Autodesk Inventor part; units mm, degrees
(part 5 of 6)
  line L1822 (91.8375, -60.1869) -> (91.8336, -60.2215) projected
  line L1823 (91.8336, -60.2215) -> (91.829, -60.2562) projected
  line L1824 (91.829, -60.2562) -> (91.8239, -60.2907) projected
  line L1825 (91.8239, -60.2907) -> (91.8181, -60.3251) projected
  line L1826 (91.8181, -60.3251) -> (91.8117, -60.3594) projected
  line L1827 (91.8117, -60.3594) -> (91.8048, -60.3936) projected
  line L1828 (91.8048, -60.3936) -> (91.7972, -60.4277) projected
  line L1829 (91.7972, -60.4277) -> (91.7891, -60.4617) projected
  line L1830 (91.7891, -60.4617) -> (91.7803, -60.4954) projected
  line L1831 (91.7803, -60.4954) -> (91.771, -60.5291) projected
  line L1832 (91.771, -60.5291) -> (91.7611, -60.5626) projected
  line L1833 (91.7611, -60.5626) -> (91.7506, -60.5958) projected
  line L1834 (91.7506, -60.5958) -> (91.7395, -60.6289) projected
  line L1835 (91.7395, -60.6289) -> (91.7279, -60.6618) projected
  line L1836 (91.7279, -60.6618) -> (91.7156, -60.6945) projected
  line L1837 (91.7156, -60.6945) -> (91.7028, -60.727) projected
  line L1838 (91.7028, -60.727) -> (91.6895, -60.7593) projected
  line L1839 (91.6895, -60.7593) -> (91.6756, -60.7913) projected
  line L1840 (91.6756, -60.7913) -> (91.6611, -60.823) projected
  line L1841 (91.6611, -60.823) -> (91.6461, -60.8546) projected
  line L1842 (91.6461, -60.8546) -> (91.6305, -60.8858) projected
  line L1843 (91.6305, -60.8858) -> (91.6144, -60.9168) projected
  line L1844 (91.6144, -60.9168) -> (91.5977, -60.9474) projected
  line L1845 (91.5977, -60.9474) -> (91.5805, -60.9778) projected
  line L1846 (91.5805, -60.9778) -> (91.5628, -61.0079) projected
  line L1847 (91.5628, -61.0079) -> (91.5446, -61.0376) projected
  line L1848 (91.5446, -61.0376) -> (91.5258, -61.0671) projected
  line L1849 (91.5258, -61.0671) -> (91.5066, -61.0962) projected
  line L1850 (91.5066, -61.0962) -> (91.4868, -61.125) projected
  line L1851 (91.4868, -61.125) -> (91.4665, -61.1534) projected
  line L1852 (91.4665, -61.1534) -> (91.4458, -61.1814) projected
  line L1853 (91.4458, -61.1814) -> (91.4245, -61.2091) projected
  line L1854 (91.4245, -61.2091) -> (91.4028, -61.2364) projected
  line L1855 (91.4028, -61.2364) -> (91.3806, -61.2634) projected
  line L1856 (91.3806, -61.2634) -> (91.3579, -61.2899) projected
  line L1857 (91.3579, -61.2899) -> (91.3348, -61.3161) projected
  line L1858 (91.3348, -61.3161) -> (91.3112, -61.3418) projected
  line L1859 (91.3112, -61.3418) -> (91.2872, -61.3671) projected
  line L1860 (91.2872, -61.3671) -> (91.2627, -61.392) projected
  line L1861 (91.2627, -61.392) -> (91.2378, -61.4165) projected
  line L1862 (91.2378, -61.4165) -> (91.2125, -61.4405) projected
  line L1863 (91.2125, -61.4405) -> (91.1867, -61.4641) projected
  line L1864 (91.1867, -61.4641) -> (91.1606, -61.4872) projected
  line L1865 (91.1606, -61.4872) -> (91.1341, -61.5099) projected
  line L1866 (91.1341, -61.5099) -> (91.1071, -61.5321) projected
  line L1867 (91.1071, -61.5321) -> (91.0798, -61.5538) projected
  line L1868 (91.0798, -61.5538) -> (91.0521, -61.5751) projected
  line L1869 (91.0521, -61.5751) -> (91.0241, -61.5958) projected
  line L1870 (91.0241, -61.5958) -> (90.9956, -61.6161) projected
  line L1871 (90.9956, -61.6161) -> (90.9669, -61.6359) projected
  line L1872 (90.9669, -61.6359) -> (90.9378, -61.6551) projected
  line L1873 (90.9378, -61.6551) -> (90.9083, -61.6739) projected
  line L1874 (90.9083, -61.6739) -> (90.8786, -61.6921) projected
  line L1875 (90.8786, -61.6921) -> (90.8485, -61.7099) projected
  line L1876 (90.8485, -61.7099) -> (90.8181, -61.727) projected
  line L1877 (90.8181, -61.727) -> (90.7874, -61.7437) projected
  line L1878 (90.7874, -61.7437) -> (90.7565, -61.7598) projected
  line L1879 (90.7565, -61.7598) -> (90.7252, -61.7754) projected
  line L1880 (90.7252, -61.7754) -> (90.6937, -61.7904) projected
  line L1881 (90.6937, -61.7904) -> (90.662, -61.8049) projected
  line L1882 (90.662, -61.8049) -> (90.6299, -61.8188) projected
  line L1883 (90.6299, -61.8188) -> (90.5977, -61.8322) projected
  line L1884 (90.5977, -61.8322) -> (90.5652, -61.845) projected
  line L1885 (90.5652, -61.845) -> (90.5325, -61.8572) projected
  line L1886 (90.5325, -61.8572) -> (90.4996, -61.8688) projected
  line L1887 (90.4996, -61.8688) -> (90.4665, -61.8799) projected
  line L1888 (90.4665, -61.8799) -> (90.4332, -61.8904) projected
  line L1889 (90.4332, -61.8904) -> (90.3998, -61.9003) projected
  line L1890 (90.3998, -61.9003) -> (90.3661, -61.9097) projected
  line L1891 (90.3661, -61.9097) -> (90.3323, -61.9184) projected
  line L1892 (90.3323, -61.9184) -> (90.2984, -61.9265) projected
  line L1893 (90.2984, -61.9265) -> (90.2643, -61.9341) projected
  line L1894 (90.2643, -61.9341) -> (90.2301, -61.9411) projected
  line L1895 (90.2301, -61.9411) -> (90.1958, -61.9474) projected
  line L1896 (90.1958, -61.9474) -> (90.1614, -61.9532) projected
  line L1897 (90.1614, -61.9532) -> (90.1268, -61.9583) projected
  line L1898 (90.1268, -61.9583) -> (90.0922, -61.9629) projected
  line L1899 (90.0922, -61.9629) -> (90.0575, -61.9668) projected
  line L1900 (90.0575, -61.9668) -> (90.0228, -61.9702) projected
  line L1901 (90.0228, -61.9702) -> (89.988, -61.9729) projected
  line L1902 (89.988, -61.9729) -> (89.9532, -61.9751) projected
  line L1903 (89.9532, -61.9751) -> (89.9183, -61.9766) projected
  line L1904 (89.9183, -61.9766) -> (89.8834, -61.9775) projected
  line L1905 (89.8834, -61.9775) -> (89.8485, -61.9778) projected
  line L1906 (89.8485, -61.9778) -> (89.8136, -61.9775) projected
  line L1907 (89.8136, -61.9775) -> (89.7787, -61.9766) projected
  line L1908 (89.7787, -61.9766) -> (89.7438, -61.9751) projected
  line L1909 (89.7438, -61.9751) -> (89.709, -61.9729) projected
  line L1910 (89.709, -61.9729) -> (89.6742, -61.9702) projected
  line L1911 (89.6742, -61.9702) -> (89.6394, -61.9668) projected
  line L1912 (89.6394, -61.9668) -> (89.6047, -61.9629) projected
  line L1913 (89.6047, -61.9629) -> (89.5701, -61.9583) projected
  line L1914 (89.5701, -61.9583) -> (89.5356, -61.9532) projected
  line L1915 (89.5356, -61.9532) -> (89.5012, -61.9474) projected
  line L1916 (89.5012, -61.9474) -> (89.4669, -61.9411) projected
  line L1917 (89.4669, -61.9411) -> (89.4327, -61.9341) projected
  line L1918 (89.4327, -61.9341) -> (89.3986, -61.9265) projected
  line L1919 (89.3986, -61.9265) -> (89.3646, -61.9184) projected
  line L1920 (89.3646, -61.9184) -> (89.3308, -61.9097) projected
  line L1921 (89.3308, -61.9097) -> (89.2972, -61.9003) projected
  line L1922 (89.2972, -61.9003) -> (89.2637, -61.8904) projected
  line L1923 (89.2637, -61.8904) -> (89.2305, -61.8799) projected
  line L1924 (89.2305, -61.8799) -> (89.1973, -61.8688) projected
  line L1925 (89.1973, -61.8688) -> (89.1644, -61.8572) projected
  line L1926 (89.1644, -61.8572) -> (89.1317, -61.845) projected
  line L1927 (89.1317, -61.845) -> (89.0993, -61.8322) projected
  line L1928 (89.0993, -61.8322) -> (89.067, -61.8188) projected
  line L1929 (89.067, -61.8188) -> (89.035, -61.8049) projected
  line L1930 (89.035, -61.8049) -> (89.0032, -61.7904) projected
  line L1931 (89.0032, -61.7904) -> (88.9717, -61.7754) projected
  line L1932 (88.9717, -61.7754) -> (88.9405, -61.7598) projected
  line L1933 (88.9405, -61.7598) -> (88.9095, -61.7437) projected
  line L1934 (88.9095, -61.7437) -> (88.8789, -61.727) projected
  line L1935 (88.8789, -61.727) -> (88.8485, -61.7099) projected
  line L1936 (88.8485, -61.7099) -> (88.8184, -61.6921) projected
  line L1937 (88.8184, -61.6921) -> (88.7886, -61.6739) projected
  line L1938 (88.7886, -61.6739) -> (88.7592, -61.6551) projected
  line L1939 (88.7592, -61.6551) -> (88.7301, -61.6359) projected
  line L1940 (88.7301, -61.6359) -> (88.7013, -61.6161) projected
  line L1941 (88.7013, -61.6161) -> (88.6729, -61.5958) projected
  line L1942 (88.6729, -61.5958) -> (88.6449, -61.5751) projected
  line L1943 (88.6449, -61.5751) -> (88.6172, -61.5538) projected
  line L1944 (88.6172, -61.5538) -> (88.5898, -61.5321) projected
  line L1945 (88.5898, -61.5321) -> (88.5629, -61.5099) projected
  line L1946 (88.5629, -61.5099) -> (88.5364, -61.4872) projected
  line L1947 (88.5364, -61.4872) -> (88.5102, -61.4641) projected
  line L1948 (88.5102, -61.4641) -> (88.4845, -61.4405) projected
  line L1949 (88.4845, -61.4405) -> (88.4592, -61.4165) projected
  line L1950 (88.4592, -61.4165) -> (88.4343, -61.392) projected
  line L1951 (88.4343, -61.392) -> (88.4098, -61.3671) projected
  line L1952 (88.4098, -61.3671) -> (88.3858, -61.3418) projected
  line L1953 (88.3858, -61.3418) -> (88.3622, -61.3161) projected
  line L1954 (88.3622, -61.3161) -> (88.3391, -61.2899) projected
  line L1955 (88.3391, -61.2899) -> (88.3164, -61.2634) projected
  line L1956 (88.3164, -61.2634) -> (88.2942, -61.2364) projected
  line L1957 (88.2942, -61.2364) -> (88.2725, -61.2091) projected
  line L1958 (88.2725, -61.2091) -> (88.2512, -61.1814) projected
  line L1959 (88.2512, -61.1814) -> (88.2305, -61.1534) projected
  line L1960 (88.2305, -61.1534) -> (88.2102, -61.125) projected
  line L1961 (88.2102, -61.125) -> (88.1904, -61.0962) projected
  line L1962 (88.1904, -61.0962) -> (88.1711, -61.0671) projected
  line L1963 (88.1711, -61.0671) -> (88.1524, -61.0376) projected
  line L1964 (88.1524, -61.0376) -> (88.1342, -61.0079) projected
  line L1965 (88.1342, -61.0079) -> (88.1164, -60.9778) projected
  line L1966 (88.1164, -60.9778) -> (88.0992, -60.9474) projected
  line L1967 (88.0992, -60.9474) -> (88.0826, -60.9168) projected
  line L1968 (88.0826, -60.9168) -> (88.0665, -60.8858) projected
  line L1969 (88.0665, -60.8858) -> (88.0509, -60.8546) projected
  line L1970 (88.0509, -60.8546) -> (88.0359, -60.823) projected
  line L1971 (88.0359, -60.823) -> (88.0214, -60.7913) projected
  line L1972 (88.0214, -60.7913) -> (88.0075, -60.7593) projected
  line L1973 (88.0075, -60.7593) -> (87.9941, -60.727) projected
  line L1974 (87.9941, -60.727) -> (87.9813, -60.6945) projected
  line L1975 (87.9813, -60.6945) -> (87.9691, -60.6618) projected
  line L1976 (87.9691, -60.6618) -> (87.9575, -60.6289) projected
  line L1977 (87.9575, -60.6289) -> (87.9464, -60.5958) projected
  line L1978 (87.9464, -60.5958) -> (87.9359, -60.5626) projected
  line L1979 (87.9359, -60.5626) -> (87.926, -60.5291) projected
  line L1980 (87.926, -60.5291) -> (87.9166, -60.4954) projected
  line L1981 (87.9166, -60.4954) -> (87.9079, -60.4617) projected
  line L1982 (87.9079, -60.4617) -> (87.8997, -60.4277) projected
  line L1983 (87.8997, -60.4277) -> (87.8922, -60.3936) projected
  line L1984 (87.8922, -60.3936) -> (87.8852, -60.3594) projected
  line L1985 (87.8852, -60.3594) -> (87.8789, -60.3251) projected
  line L1986 (87.8789, -60.3251) -> (87.8731, -60.2907) projected
  line L1987 (87.8731, -60.2907) -> (87.868, -60.2562) projected
  line L1988 (87.868, -60.2562) -> (87.8634, -60.2215) projected
  line L1989 (87.8634, -60.2215) -> (87.8594, -60.1869) projected
  line L1990 (87.8594, -60.1869) -> (87.8561, -60.1521) projected
  line L1991 (87.8561, -60.1521) -> (87.8534, -60.1173) projected
  line L1992 (87.8534, -60.1173) -> (87.8512, -60.0825) projected
  line L1993 (87.8512, -60.0825) -> (87.8497, -60.0476) projected
  line L1994 (87.8497, -60.0476) -> (87.8488, -60.0127) projected
  line L1995 (87.8488, -60.0127) -> (87.8485, -59.9778) projected
  line L1996 (87.8485, -59.9778) -> (87.8488, -59.9429) projected
  line L1997 (87.8488, -59.9429) -> (87.8497, -59.908) projected
  line L1998 (87.8497, -59.908) -> (87.8512, -59.8731) projected
  line L1999 (87.8512, -59.8731) -> (87.8534, -59.8383) projected
  line L2000 (87.8534, -59.8383) -> (87.8561, -59.8035) projected
  line L2001 (87.8561, -59.8035) -> (87.8594, -59.7688) projected
  line L2002 (87.8594, -59.7688) -> (87.8634, -59.7341) projected
  line L2003 (87.8634, -59.7341) -> (87.868, -59.6995) projected
  line L2004 (87.868, -59.6995) -> (87.8731, -59.6649) projected
  line L2005 (87.8731, -59.6649) -> (87.8789, -59.6305) projected
  line L2006 (87.8789, -59.6305) -> (87.8852, -59.5962) projected
  line L2007 (87.8852, -59.5962) -> (87.8922, -59.562) projected
  line L2008 (87.8922, -59.562) -> (87.8997, -59.5279) projected
  line L2009 (87.8997, -59.5279) -> (87.9079, -59.494) projected
  line L2010 (87.9079, -59.494) -> (87.9166, -59.4602) projected
  line L2011 (87.9166, -59.4602) -> (87.926, -59.4265) projected
  line L2012 (87.926, -59.4265) -> (87.9359, -59.3931) projected
  line L2013 (87.9359, -59.3931) -> (87.9464, -59.3598) projected
  line L2014 (87.9464, -59.3598) -> (87.9575, -59.3267) projected
  line L2015 (87.9575, -59.3267) -> (87.9691, -59.2938) projected
  line L2016 (87.9691, -59.2938) -> (87.9813, -59.2611) projected
  line L2017 (87.9813, -59.2611) -> (87.9941, -59.2286) projected
  line L2018 (87.9941, -59.2286) -> (88.0075, -59.1963) projected
  line L2019 (88.0075, -59.1963) -> (88.0214, -59.1643) projected
  line L2020 (88.0214, -59.1643) -> (88.0359, -59.1326) projected
  line L2021 (88.0359, -59.1326) -> (88.0509, -59.1011) projected
  line L2022 (88.0509, -59.1011) -> (88.0665, -59.0698) projected
  line L2023 (88.0665, -59.0698) -> (88.0826, -59.0389) projected
  line L2024 (88.0826, -59.0389) -> (88.0992, -59.0082) projected
  line L2025 (88.0992, -59.0082) -> (88.1164, -58.9778) projected
  line L2026 (88.1164, -58.9778) -> (88.1342, -58.9477) projected
  line L2027 (88.1342, -58.9477) -> (88.1524, -58.918) projected
  line L2028 (88.1524, -58.918) -> (88.1711, -58.8885) projected
  line L2029 (88.1711, -58.8885) -> (88.1904, -58.8594) projected
  line L2030 (88.1904, -58.8594) -> (88.2102, -58.8307) projected
  line L2031 (88.2102, -58.8307) -> (88.2305, -58.8022) projected
  line L2032 (88.2305, -58.8022) -> (88.2512, -58.7742) projected
  line L2033 (88.2512, -58.7742) -> (88.2725, -58.7465) projected
  line L2034 (88.2725, -58.7465) -> (88.2942, -58.7192) projected
  line L2035 (88.2942, -58.7192) -> (88.3164, -58.6922) projected
  line L2036 (88.3164, -58.6922) -> (88.3391, -58.6657) projected
  line L2037 (88.3391, -58.6657) -> (88.3622, -58.6396) projected
  line L2038 (88.3622, -58.6396) -> (88.3858, -58.6138) projected
  line L2039 (88.3858, -58.6138) -> (88.4098, -58.5885) projected
  line L2040 (88.4098, -58.5885) -> (88.4343, -58.5636) projected
  line L2041 (88.4343, -58.5636) -> (88.4592, -58.5391) projected
  line L2042 (88.4592, -58.5391) -> (88.4845, -58.5151) projected
  line L2043 (88.4845, -58.5151) -> (88.5102, -58.4915) projected
  line L2044 (88.5102, -58.4915) -> (88.5364, -58.4684) projected
  line L2045 (88.5364, -58.4684) -> (88.5629, -58.4457) projected
  line L2046 (88.5629, -58.4457) -> (88.5898, -58.4235) projected
  line L2047 (88.5898, -58.4235) -> (88.6172, -58.4018) projected
  line L2048 (88.6172, -58.4018) -> (88.6449, -58.3805) projected
  line L2049 (88.6449, -58.3805) -> (88.6729, -58.3598) projected
  line L2050 (88.6729, -58.3598) -> (88.7013, -58.3395) projected
  line L2051 (88.7013, -58.3395) -> (88.7301, -58.3197) projected
  line L2052 (88.7301, -58.3197) -> (88.7592, -58.3005) projected
  line L2053 (88.7592, -58.3005) -> (88.7886, -58.2817) projected
  line L2054 (88.7886, -58.2817) -> (88.8184, -58.2635) projected
  line L2055 (88.8184, -58.2635) -> (88.8485, -58.2458) projected
  line L2056 (88.8485, -58.2458) -> (88.8789, -58.2286) projected
  line L2057 (88.8789, -58.2286) -> (88.9095, -58.2119) projected
  line L2058 (88.9095, -58.2119) -> (88.9405, -58.1958) projected
  line L2059 (88.9405, -58.1958) -> (88.9717, -58.1802) projected
  line L2060 (88.9717, -58.1802) -> (89.0032, -58.1652) projected
  line L2061 (89.0032, -58.1652) -> (89.035, -58.1507) projected
  line L2062 (89.035, -58.1507) -> (89.067, -58.1368) projected
  line L2063 (89.067, -58.1368) -> (89.0993, -58.1234) projected
  line L2064 (89.0993, -58.1234) -> (89.1317, -58.1107) projected
  line L2065 (89.1317, -58.1107) -> (89.1644, -58.0984) projected
  line L2066 (89.1644, -58.0984) -> (89.1973, -58.0868) projected
  line L2067 (89.1973, -58.0868) -> (89.2305, -58.0757) projected
  line L2068 (89.2305, -58.0757) -> (89.2637, -58.0652) projected
  line L2069 (89.2637, -58.0652) -> (89.2972, -58.0553) projected
  line L2070 (89.2972, -58.0553) -> (89.3308, -58.046) projected
  line L2071 (89.3308, -58.046) -> (89.3646, -58.0372) projected
  line L2072 (89.3646, -58.0372) -> (89.3986, -58.0291) projected
  line L2073 (89.3986, -58.0291) -> (89.4327, -58.0215) projected
  line L2074 (89.4327, -58.0215) -> (89.4669, -58.0146) projected
  line L2075 (89.4669, -58.0146) -> (89.5012, -58.0082) projected
  line L2076 (89.5012, -58.0082) -> (89.5356, -58.0024) projected
  line L2077 (89.5356, -58.0024) -> (89.5701, -57.9973) projected
  line L2078 (89.5701, -57.9973) -> (89.6047, -57.9927) projected
  line L2079 (89.6047, -57.9927) -> (89.6394, -57.9888) projected
  line L2080 (89.6394, -57.9888) -> (89.6742, -57.9854) projected
  line L2081 (89.6742, -57.9854) -> (89.709, -57.9827) projected
  line L2082 (89.709, -57.9827) -> (89.7438, -57.9806) projected
  line L2083 (89.7438, -57.9806) -> (89.7787, -57.979) projected
  line L2084 (89.7787, -57.979) -> (89.8136, -57.9781) projected
  line L2085 (89.8136, -57.9781) -> (89.8485, -57.9778) projected
  line L2086 (89.8485, -57.9778) -> (89.8834, -57.9781) projected
  line L2087 (89.8834, -57.9781) -> (89.9183, -57.979) projected
  line L2088 (89.9183, -57.979) -> (89.9532, -57.9806) projected
  line L2089 (89.9532, -57.9806) -> (89.988, -57.9827) projected
  line L2090 (89.988, -57.9827) -> (90.0228, -57.9854) projected
  line L2091 (90.0228, -57.9854) -> (90.0575, -57.9888) projected
  line L2092 (90.0575, -57.9888) -> (90.0922, -57.9927) projected
  line L2093 (90.0922, -57.9927) -> (90.1268, -57.9973) projected
  line L2094 (90.1268, -57.9973) -> (90.1614, -58.0024) projected
  line L2095 (90.1614, -58.0024) -> (90.1958, -58.0082) projected
  line L2096 (90.1958, -58.0082) -> (90.2301, -58.0146) projected
  line L2097 (90.2301, -58.0146) -> (90.2643, -58.0215) projected
  line L2098 (90.2643, -58.0215) -> (90.2984, -58.0291) projected
  line L2099 (90.2984, -58.0291) -> (90.3323, -58.0372) projected
  line L2100 (90.3323, -58.0372) -> (90.3661, -58.046) projected
  line L2101 (90.3661, -58.046) -> (90.3998, -58.0553) projected
  line L2102 (90.3998, -58.0553) -> (90.4332, -58.0652) projected
  line L2103 (90.4332, -58.0652) -> (90.4665, -58.0757) projected
  line L2104 (90.4665, -58.0757) -> (90.4996, -58.0868) projected
  line L2105 (90.4996, -58.0868) -> (90.5325, -58.0984) projected
  line L2106 (90.5325, -58.0984) -> (90.5652, -58.1107) projected
  line L2107 (90.5652, -58.1107) -> (90.5977, -58.1234) projected
  line L2108 (90.5977, -58.1234) -> (90.6299, -58.1368) projected
  line L2109 (90.6299, -58.1368) -> (90.662, -58.1507) projected
  line L2110 (90.662, -58.1507) -> (90.6937, -58.1652) projected
  line L2111 (90.6937, -58.1652) -> (90.7252, -58.1802) projected
  line L2112 (90.7252, -58.1802) -> (90.7565, -58.1958) projected
  line L2113 (90.7565, -58.1958) -> (90.7874, -58.2119) projected
  line L2114 (90.7874, -58.2119) -> (90.8181, -58.2286) projected
  line L2115 (90.8181, -58.2286) -> (90.8485, -58.2458) projected
  line L2116 (90.8485, -58.2458) -> (90.8786, -58.2635) projected
  line L2117 (90.8786, -58.2635) -> (90.9083, -58.2817) projected
  line L2118 (90.9083, -58.2817) -> (90.9378, -58.3005) projected
  line L2119 (90.9378, -58.3005) -> (90.9669, -58.3197) projected
  line L2120 (90.9669, -58.3197) -> (90.9956, -58.3395) projected
  line L2121 (90.9956, -58.3395) -> (91.0241, -58.3598) projected
  line L2122 (91.0241, -58.3598) -> (91.0521, -58.3805) projected
  line L2123 (91.0521, -58.3805) -> (91.0798, -58.4018) projected
  line L2124 (91.0798, -58.4018) -> (91.1071, -58.4235) projected
  line L2125 (91.1071, -58.4235) -> (91.1341, -58.4457) projected
  line L2126 (91.1341, -58.4457) -> (91.1606, -58.4684) projected
  line L2127 (91.1606, -58.4684) -> (91.1867, -58.4915) projected
  line L2128 (91.1867, -58.4915) -> (91.2125, -58.5151) projected
  line L2129 (91.2125, -58.5151) -> (91.2378, -58.5391) projected
  line L2130 (91.2378, -58.5391) -> (91.2627, -58.5636) projected
  line L2131 (91.2627, -58.5636) -> (91.2872, -58.5885) projected
  line L2132 (91.2872, -58.5885) -> (91.3112, -58.6138) projected
  line L2133 (91.3112, -58.6138) -> (91.3348, -58.6396) projected
  line L2134 (91.3348, -58.6396) -> (91.3579, -58.6657) projected
  line L2135 (91.3579, -58.6657) -> (91.3806, -58.6922) projected
  line L2136 (91.3806, -58.6922) -> (91.4028, -58.7192) projected
  line L2137 (91.4028, -58.7192) -> (91.4245, -58.7465) projected
  line L2138 (91.4245, -58.7465) -> (91.4458, -58.7742) projected
  line L2139 (91.4458, -58.7742) -> (91.4665, -58.8022) projected
  line L2140 (91.4665, -58.8022) -> (91.4868, -58.8307) projected
  line L2141 (91.4868, -58.8307) -> (91.5066, -58.8594) projected
  line L2142 (91.5066, -58.8594) -> (91.5258, -58.8885) projected
  line L2143 (91.5258, -58.8885) -> (91.5446, -58.918) projected
  line L2144 (91.5446, -58.918) -> (91.5628, -58.9477) projected
  line L2145 (91.5628, -58.9477) -> (91.5805, -58.9778) projected
  line L2146 (91.5805, -58.9778) -> (91.5977, -59.0082) projected
  line L2147 (91.5977, -59.0082) -> (91.6144, -59.0389) projected
  line L2148 (91.6144, -59.0389) -> (91.6305, -59.0698) projected
  line L2149 (91.6305, -59.0698) -> (91.6461, -59.1011) projected
  line L2150 (91.6461, -59.1011) -> (91.6611, -59.1326) projected
  line L2151 (91.6611, -59.1326) -> (91.6756, -59.1643) projected
  line L2152 (91.6756, -59.1643) -> (91.6895, -59.1963) projected
  line L2153 (91.6895, -59.1963) -> (91.7028, -59.2286) projected
  line L2154 (91.7028, -59.2286) -> (91.7156, -59.2611) projected
  line L2155 (91.7156, -59.2611) -> (91.7279, -59.2938) projected
  line L2156 (91.7279, -59.2938) -> (91.7395, -59.3267) projected
  line L2157 (91.7395, -59.3267) -> (91.7506, -59.3598) projected
  line L2158 (91.7506, -59.3598) -> (91.7611, -59.3931) projected
  line L2159 (91.7611, -59.3931) -> (91.771, -59.4265) projected
  line L2160 (91.771, -59.4265) -> (91.7803, -59.4602) projected
  line L2161 (91.7803, -59.4602) -> (91.7891, -59.494) projected
  line L2162 (91.7891, -59.494) -> (91.7972, -59.5279) projected
  line L2163 (91.7972, -59.5279) -> (91.8048, -59.562) projected
  line L2164 (91.8048, -59.562) -> (91.8117, -59.5962) projected
  line L2165 (91.8117, -59.5962) -> (91.8181, -59.6305) projected
  line L2166 (91.8181, -59.6305) -> (91.8239, -59.6649) projected
  line L2167 (91.8239, -59.6649) -> (91.829, -59.6995) projected
  line L2168 (91.829, -59.6995) -> (91.8336, -59.7341) projected
  line L2169 (91.8336, -59.7341) -> (91.8375, -59.7688) projected
  line L2170 (91.8375, -59.7688) -> (91.8409, -59.8035) projected
  line L2171 (91.8409, -59.8035) -> (91.8436, -59.8383) projected
  line L2172 (91.8436, -59.8383) -> (91.8457, -59.8731) projected
  line L2173 (91.8457, -59.8731) -> (91.8473, -59.908) projected
  line L2174 (91.8473, -59.908) -> (91.8482, -59.9429) projected
  line L2175 (91.8482, -59.9429) -> (91.8485, -59.9778) projected
  line L2176 (-88.1514, -59.9778) -> (-88.1517, -60.0127) projected
  line L2177 (-88.1517, -60.0127) -> (-88.1526, -60.0476) projected
  line L2178 (-88.1526, -60.0476) -> (-88.1542, -60.0825) projected
  line L2179 (-88.1542, -60.0825) -> (-88.1563, -60.1173) projected
  line L2180 (-88.1563, -60.1173) -> (-88.159, -60.1521) projected
  line L2181 (-88.159, -60.1521) -> (-88.1624, -60.1869) projected
  line L2182 (-88.1624, -60.1869) -> (-88.1663, -60.2215) projected
  line L2183 (-88.1663, -60.2215) -> (-88.1709, -60.2562) projected
  line L2184 (-88.1709, -60.2562) -> (-88.176, -60.2907) projected
  line L2185 (-88.176, -60.2907) -> (-88.1818, -60.3251) projected
  line L2186 (-88.1818, -60.3251) -> (-88.1882, -60.3594) projected
  line L2187 (-88.1882, -60.3594) -> (-88.1951, -60.3936) projected
  line L2188 (-88.1951, -60.3936) -> (-88.2027, -60.4277) projected
  line L2189 (-88.2027, -60.4277) -> (-88.2108, -60.4617) projected
  line L2190 (-88.2108, -60.4617) -> (-88.2196, -60.4954) projected
  line L2191 (-88.2196, -60.4954) -> (-88.2289, -60.5291) projected
  line L2192 (-88.2289, -60.5291) -> (-88.2388, -60.5626) projected
  line L2193 (-88.2388, -60.5626) -> (-88.2493, -60.5958) projected
  line L2194 (-88.2493, -60.5958) -> (-88.2604, -60.6289) projected
  line L2195 (-88.2604, -60.6289) -> (-88.272, -60.6618) projected
  line L2196 (-88.272, -60.6618) -> (-88.2843, -60.6945) projected
  line L2197 (-88.2843, -60.6945) -> (-88.297, -60.727) projected
  line L2198 (-88.297, -60.727) -> (-88.3104, -60.7593) projected
  line L2199 (-88.3104, -60.7593) -> (-88.3243, -60.7913) projected
  line L2200 (-88.3243, -60.7913) -> (-88.3388, -60.823) projected
  line L2201 (-88.3388, -60.823) -> (-88.3538, -60.8546) projected
  line L2202 (-88.3538, -60.8546) -> (-88.3694, -60.8858) projected
  line L2203 (-88.3694, -60.8858) -> (-88.3855, -60.9168) projected
  line L2204 (-88.3855, -60.9168) -> (-88.4022, -60.9474) projected
  line L2205 (-88.4022, -60.9474) -> (-88.4194, -60.9778) projected
  line L2206 (-88.4194, -60.9778) -> (-88.4371, -61.0079) projected
  line L2207 (-88.4371, -61.0079) -> (-88.4553, -61.0376) projected
  line L2208 (-88.4553, -61.0376) -> (-88.4741, -61.0671) projected
  line L2209 (-88.4741, -61.0671) -> (-88.4933, -61.0962) projected
  line L2210 (-88.4933, -61.0962) -> (-88.5131, -61.125) projected
  line L2211 (-88.5131, -61.125) -> (-88.5334, -61.1534) projected
  line L2212 (-88.5334, -61.1534) -> (-88.5541, -61.1814) projected
  line L2213 (-88.5541, -61.1814) -> (-88.5754, -61.2091) projected
  line L2214 (-88.5754, -61.2091) -> (-88.5971, -61.2364) projected
  line L2215 (-88.5971, -61.2364) -> (-88.6193, -61.2634) projected
  line L2216 (-88.6193, -61.2634) -> (-88.642, -61.2899) projected
  line L2217 (-88.642, -61.2899) -> (-88.6651, -61.3161) projected
  line L2218 (-88.6651, -61.3161) -> (-88.6887, -61.3418) projected
  line L2219 (-88.6887, -61.3418) -> (-88.7127, -61.3671) projected
  line L2220 (-88.7127, -61.3671) -> (-88.7372, -61.392) projected
  line L2221 (-88.7372, -61.392) -> (-88.7621, -61.4165) projected
  line L2222 (-88.7621, -61.4165) -> (-88.7874, -61.4405) projected
  line L2223 (-88.7874, -61.4405) -> (-88.8132, -61.4641) projected
  line L2224 (-88.8132, -61.4641) -> (-88.8393, -61.4872) projected
  line L2225 (-88.8393, -61.4872) -> (-88.8658, -61.5099) projected
  line L2226 (-88.8658, -61.5099) -> (-88.8928, -61.5321) projected
  line L2227 (-88.8928, -61.5321) -> (-88.9201, -61.5538) projected
  line L2228 (-88.9201, -61.5538) -> (-88.9478, -61.5751) projected
  line L2229 (-88.9478, -61.5751) -> (-88.9758, -61.5958) projected
  line L2230 (-88.9758, -61.5958) -> (-89.0043, -61.6161) projected
  line L2231 (-89.0043, -61.6161) -> (-89.033, -61.6359) projected
  line L2232 (-89.033, -61.6359) -> (-89.0621, -61.6551) projected
  line L2233 (-89.0621, -61.6551) -> (-89.0916, -61.6739) projected
  line L2234 (-89.0916, -61.6739) -> (-89.1213, -61.6921) projected
  line L2235 (-89.1213, -61.6921) -> (-89.1514, -61.7099) projected
  line L2236 (-89.1514, -61.7099) -> (-89.1818, -61.727) projected
  line L2237 (-89.1818, -61.727) -> (-89.2125, -61.7437) projected
  line L2238 (-89.2125, -61.7437) -> (-89.2434, -61.7598) projected
  line L2239 (-89.2434, -61.7598) -> (-89.2747, -61.7754) projected
  line L2240 (-89.2747, -61.7754) -> (-89.3062, -61.7904) projected
  line L2241 (-89.3062, -61.7904) -> (-89.3379, -61.8049) projected
  line L2242 (-89.3379, -61.8049) -> (-89.3699, -61.8188) projected
  line L2243 (-89.3699, -61.8188) -> (-89.4022, -61.8322) projected
  line L2244 (-89.4022, -61.8322) -> (-89.4347, -61.845) projected
  line L2245 (-89.4347, -61.845) -> (-89.4674, -61.8572) projected
  line L2246 (-89.4674, -61.8572) -> (-89.5003, -61.8688) projected
  line L2247 (-89.5003, -61.8688) -> (-89.5334, -61.8799) projected
  line L2248 (-89.5334, -61.8799) -> (-89.5667, -61.8904) projected
  line L2249 (-89.5667, -61.8904) -> (-89.6001, -61.9003) projected
  line L2250 (-89.6001, -61.9003) -> (-89.6338, -61.9097) projected
  line L2251 (-89.6338, -61.9097) -> (-89.6676, -61.9184) projected
  line L2252 (-89.6676, -61.9184) -> (-89.7015, -61.9265) projected
  line L2253 (-89.7015, -61.9265) -> (-89.7356, -61.9341) projected
  line L2254 (-89.7356, -61.9341) -> (-89.7698, -61.9411) projected
  line L2255 (-89.7698, -61.9411) -> (-89.8041, -61.9474) projected
  line L2256 (-89.8041, -61.9474) -> (-89.8385, -61.9532) projected
  line L2257 (-89.8385, -61.9532) -> (-89.8731, -61.9583) projected
  line L2258 (-89.8731, -61.9583) -> (-89.9077, -61.9629) projected
  line L2259 (-89.9077, -61.9629) -> (-89.9424, -61.9668) projected
  line L2260 (-89.9424, -61.9668) -> (-89.9771, -61.9702) projected
  line L2261 (-89.9771, -61.9702) -> (-90.0119, -61.9729) projected
  line L2262 (-90.0119, -61.9729) -> (-90.0467, -61.9751) projected
  line L2263 (-90.0467, -61.9751) -> (-90.0816, -61.9766) projected
  line L2264 (-90.0816, -61.9766) -> (-90.1165, -61.9775) projected
  line L2265 (-90.1165, -61.9775) -> (-90.1514, -61.9778) projected
  line L2266 (-90.1514, -61.9778) -> (-90.1863, -61.9775) projected
  line L2267 (-90.1863, -61.9775) -> (-90.2212, -61.9766) projected
  line L2268 (-90.2212, -61.9766) -> (-90.2561, -61.9751) projected
  line L2269 (-90.2561, -61.9751) -> (-90.2909, -61.9729) projected
  line L2270 (-90.2909, -61.9729) -> (-90.3257, -61.9702) projected
  line L2271 (-90.3257, -61.9702) -> (-90.3605, -61.9668) projected
  line L2272 (-90.3605, -61.9668) -> (-90.3951, -61.9629) projected
  line L2273 (-90.3951, -61.9629) -> (-90.4298, -61.9583) projected
  line L2274 (-90.4298, -61.9583) -> (-90.4643, -61.9532) projected
  line L2275 (-90.4643, -61.9532) -> (-90.4987, -61.9474) projected
  line L2276 (-90.4987, -61.9474) -> (-90.533, -61.9411) projected
  line L2277 (-90.533, -61.9411) -> (-90.5672, -61.9341) projected
  line L2278 (-90.5672, -61.9341) -> (-90.6013, -61.9265) projected
  line L2279 (-90.6013, -61.9265) -> (-90.6353, -61.9184) projected
  line L2280 (-90.6353, -61.9184) -> (-90.669, -61.9097) projected
  line L2281 (-90.669, -61.9097) -> (-90.7027, -61.9003) projected
  line L2282 (-90.7027, -61.9003) -> (-90.7362, -61.8904) projected
  line L2283 (-90.7362, -61.8904) -> (-90.7694, -61.8799) projected
  line L2284 (-90.7694, -61.8799) -> (-90.8025, -61.8688) projected
  line L2285 (-90.8025, -61.8688) -> (-90.8354, -61.8572) projected
  line L2286 (-90.8354, -61.8572) -> (-90.8681, -61.845) projected
  line L2287 (-90.8681, -61.845) -> (-90.9006, -61.8322) projected
  line L2288 (-90.9006, -61.8322) -> (-90.9329, -61.8188) projected
  line L2289 (-90.9329, -61.8188) -> (-90.9649, -61.8049) projected
  line L2290 (-90.9649, -61.8049) -> (-90.9966, -61.7904) projected
  line L2291 (-90.9966, -61.7904) -> (-91.0282, -61.7754) projected
  line L2292 (-91.0282, -61.7754) -> (-91.0594, -61.7598) projected
  line L2293 (-91.0594, -61.7598) -> (-91.0904, -61.7437) projected
  line L2294 (-91.0904, -61.7437) -> (-91.121, -61.727) projected
  line L2295 (-91.121, -61.727) -> (-91.1514, -61.7099) projected
  line L2296 (-91.1514, -61.7099) -> (-91.1815, -61.6921) projected
  line L2297 (-91.1815, -61.6921) -> (-91.2112, -61.6739) projected
  line L2298 (-91.2112, -61.6739) -> (-91.2407, -61.6551) projected
  line L2299 (-91.2407, -61.6551) -> (-91.2698, -61.6359) projected
  line L2300 (-91.2698, -61.6359) -> (-91.2986, -61.6161) projected
  line L2301 (-91.2986, -61.6161) -> (-91.327, -61.5958) projected
  line L2302 (-91.327, -61.5958) -> (-91.355, -61.5751) projected
  line L2303 (-91.355, -61.5751) -> (-91.3827, -61.5538) projected
  line L2304 (-91.3827, -61.5538) -> (-91.41, -61.5321) projected
  line L2305 (-91.41, -61.5321) -> (-91.437, -61.5099) projected
  line L2306 (-91.437, -61.5099) -> (-91.4635, -61.4872) projected
  line L2307 (-91.4635, -61.4872) -> (-91.4897, -61.4641) projected
  line L2308 (-91.4897, -61.4641) -> (-91.5154, -61.4405) projected
  line L2309 (-91.5154, -61.4405) -> (-91.5407, -61.4165) projected
  line L2310 (-91.5407, -61.4165) -> (-91.5656, -61.392) projected
  line L2311 (-91.5656, -61.392) -> (-91.5901, -61.3671) projected
  line L2312 (-91.5901, -61.3671) -> (-91.6141, -61.3418) projected
  line L2313 (-91.6141, -61.3418) -> (-91.6377, -61.3161) projected
  line L2314 (-91.6377, -61.3161) -> (-91.6608, -61.2899) projected
  line L2315 (-91.6608, -61.2899) -> (-91.6835, -61.2634) projected
  line L2316 (-91.6835, -61.2634) -> (-91.7057, -61.2364) projected
  line L2317 (-91.7057, -61.2364) -> (-91.7274, -61.2091) projected
  line L2318 (-91.7274, -61.2091) -> (-91.7487, -61.1814) projected
  line L2319 (-91.7487, -61.1814) -> (-91.7694, -61.1534) projected
  line L2320 (-91.7694, -61.1534) -> (-91.7897, -61.125) projected
  line L2321 (-91.7897, -61.125) -> (-91.8095, -61.0962) projected
  line L2322 (-91.8095, -61.0962) -> (-91.8287, -61.0671) projected
  line L2323 (-91.8287, -61.0671) -> (-91.8475, -61.0376) projected
  line L2324 (-91.8475, -61.0376) -> (-91.8657, -61.0079) projected
  line L2325 (-91.8657, -61.0079) -> (-91.8835, -60.9778) projected
  line L2326 (-91.8835, -60.9778) -> (-91.9006, -60.9474) projected
  line L2327 (-91.9006, -60.9474) -> (-91.9173, -60.9168) projected
  line L2328 (-91.9173, -60.9168) -> (-91.9334, -60.8858) projected
  line L2329 (-91.9334, -60.8858) -> (-91.949, -60.8546) projected
  line L2330 (-91.949, -60.8546) -> (-91.964, -60.823) projected
  line L2331 (-91.964, -60.823) -> (-91.9785, -60.7913) projected
  line L2332 (-91.9785, -60.7913) -> (-91.9924, -60.7593) projected
  line L2333 (-91.9924, -60.7593) -> (-92.0058, -60.727) projected
  line L2334 (-92.0058, -60.727) -> (-92.0186, -60.6945) projected
  line L2335 (-92.0186, -60.6945) -> (-92.0308, -60.6618) projected
  line L2336 (-92.0308, -60.6618) -> (-92.0424, -60.6289) projected
  line L2337 (-92.0424, -60.6289) -> (-92.0535, -60.5958) projected
  line L2338 (-92.0535, -60.5958) -> (-92.064, -60.5626) projected
  line L2339 (-92.064, -60.5626) -> (-92.0739, -60.5291) projected
  line L2340 (-92.0739, -60.5291) -> (-92.0833, -60.4954) projected
  line L2341 (-92.0833, -60.4954) -> (-92.092, -60.4617) projected
  line L2342 (-92.092, -60.4617) -> (-92.1001, -60.4277) projected
  line L2343 (-92.1001, -60.4277) -> (-92.1077, -60.3936) projected
  line L2344 (-92.1077, -60.3936) -> (-92.1147, -60.3594) projected
  line L2345 (-92.1147, -60.3594) -> (-92.121, -60.3251) projected
  line L2346 (-92.121, -60.3251) -> (-92.1268, -60.2907) projected
  line L2347 (-92.1268, -60.2907) -> (-92.1319, -60.2562) projected
  line L2348 (-92.1319, -60.2562) -> (-92.1365, -60.2215) projected
  line L2349 (-92.1365, -60.2215) -> (-92.1404, -60.1869) projected
  line L2350 (-92.1404, -60.1869) -> (-92.1438, -60.1521) projected
  line L2351 (-92.1438, -60.1521) -> (-92.1465, -60.1173) projected
  line L2352 (-92.1465, -60.1173) -> (-92.1487, -60.0825) projected
  line L2353 (-92.1487, -60.0825) -> (-92.1502, -60.0476) projected
  line L2354 (-92.1502, -60.0476) -> (-92.1511, -60.0127) projected
  line L2355 (-92.1511, -60.0127) -> (-92.1514, -59.9778) projected
  line L2356 (-92.1514, -59.9778) -> (-92.1511, -59.9429) projected
  line L2357 (-92.1511, -59.9429) -> (-92.1502, -59.908) projected
  line L2358 (-92.1502, -59.908) -> (-92.1487, -59.8731) projected
  line L2359 (-92.1487, -59.8731) -> (-92.1465, -59.8383) projected
  line L2360 (-92.1465, -59.8383) -> (-92.1438, -59.8035) projected
  line L2361 (-92.1438, -59.8035) -> (-92.1404, -59.7688) projected
  line L2362 (-92.1404, -59.7688) -> (-92.1365, -59.7341) projected
  line L2363 (-92.1365, -59.7341) -> (-92.1319, -59.6995) projected
  line L2364 (-92.1319, -59.6995) -> (-92.1268, -59.6649) projected
  line L2365 (-92.1268, -59.6649) -> (-92.121, -59.6305) projected
  line L2366 (-92.121, -59.6305) -> (-92.1147, -59.5962) projected
  line L2367 (-92.1147, -59.5962) -> (-92.1077, -59.562) projected
  line L2368 (-92.1077, -59.562) -> (-92.1001, -59.5279) projected
  line L2369 (-92.1001, -59.5279) -> (-92.092, -59.494) projected
  line L2370 (-92.092, -59.494) -> (-92.0833, -59.4602) projected
  line L2371 (-92.0833, -59.4602) -> (-92.0739, -59.4265) projected
  line L2372 (-92.0739, -59.4265) -> (-92.064, -59.3931) projected
  line L2373 (-92.064, -59.3931) -> (-92.0535, -59.3598) projected
  line L2374 (-92.0535, -59.3598) -> (-92.0424, -59.3267) projected
  line L2375 (-92.0424, -59.3267) -> (-92.0308, -59.2938) projected
  line L2376 (-92.0308, -59.2938) -> (-92.0186, -59.2611) projected
  line L2377 (-92.0186, -59.2611) -> (-92.0058, -59.2286) projected
  line L2378 (-92.0058, -59.2286) -> (-91.9924, -59.1963) projected
  line L2379 (-91.9924, -59.1963) -> (-91.9785, -59.1643) projected
  line L2380 (-91.9785, -59.1643) -> (-91.964, -59.1326) projected
  line L2381 (-91.964, -59.1326) -> (-91.949, -59.1011) projected
  line L2382 (-91.949, -59.1011) -> (-91.9334, -59.0698) projected
  line L2383 (-91.9334, -59.0698) -> (-91.9173, -59.0389) projected
  line L2384 (-91.9173, -59.0389) -> (-91.9006, -59.0082) projected
  line L2385 (-91.9006, -59.0082) -> (-91.8835, -58.9778) projected
  line L2386 (-91.8835, -58.9778) -> (-91.8657, -58.9477) projected
  line L2387 (-91.8657, -58.9477) -> (-91.8475, -58.918) projected
  line L2388 (-91.8475, -58.918) -> (-91.8287, -58.8885) projected
  line L2389 (-91.8287, -58.8885) -> (-91.8095, -58.8594) projected
  line L2390 (-91.8095, -58.8594) -> (-91.7897, -58.8307) projected
  line L2391 (-91.7897, -58.8307) -> (-91.7694, -58.8022) projected
  line L2392 (-91.7694, -58.8022) -> (-91.7487, -58.7742) projected
  line L2393 (-91.7487, -58.7742) -> (-91.7274, -58.7465) projected
  line L2394 (-91.7274, -58.7465) -> (-91.7057, -58.7192) projected
  line L2395 (-91.7057, -58.7192) -> (-91.6835, -58.6922) projected
  line L2396 (-91.6835, -58.6922) -> (-91.6608, -58.6657) projected
  line L2397 (-91.6608, -58.6657) -> (-91.6377, -58.6396) projected
  line L2398 (-91.6377, -58.6396) -> (-91.6141, -58.6138) projected
  line L2399 (-91.6141, -58.6138) -> (-91.5901, -58.5885) projected
  line L2400 (-91.5901, -58.5885) -> (-91.5656, -58.5636) projected
  line L2401 (-91.5656, -58.5636) -> (-91.5407, -58.5391) projected
  line L2402 (-91.5407, -58.5391) -> (-91.5154, -58.5151) projected
  line L2403 (-91.5154, -58.5151) -> (-91.4897, -58.4915) projected
  line L2404 (-91.4897, -58.4915) -> (-91.4635, -58.4684) projected
  line L2405 (-91.4635, -58.4684) -> (-91.437, -58.4457) projected
  line L2406 (-91.437, -58.4457) -> (-91.41, -58.4235) projected
  line L2407 (-91.41, -58.4235) -> (-91.3827, -58.4018) projected
  line L2408 (-91.3827, -58.4018) -> (-91.355, -58.3805) projected
  line L2409 (-91.355, -58.3805) -> (-91.327, -58.3598) projected
  line L2410 (-91.327, -58.3598) -> (-91.2986, -58.3395) projected
  line L2411 (-91.2986, -58.3395) -> (-91.2698, -58.3197) projected
  line L2412 (-91.2698, -58.3197) -> (-91.2407, -58.3005) projected
  line L2413 (-91.2407, -58.3005) -> (-91.2112, -58.2817) projected
  line L2414 (-91.2112, -58.2817) -> (-91.1815, -58.2635) projected
  line L2415 (-91.1815, -58.2635) -> (-91.1514, -58.2458) projected
  line L2416 (-91.1514, -58.2458) -> (-91.121, -58.2286) projected
  line L2417 (-91.121, -58.2286) -> (-91.0904, -58.2119) projected
  line L2418 (-91.0904, -58.2119) -> (-91.0594, -58.1958) projected
  line L2419 (-91.0594, -58.1958) -> (-91.0282, -58.1802) projected
  line L2420 (-91.0282, -58.1802) -> (-90.9966, -58.1652) projected
  line L2421 (-90.9966, -58.1652) -> (-90.9649, -58.1507) projected
  line L2422 (-90.9649, -58.1507) -> (-90.9329, -58.1368) projected
  line L2423 (-90.9329, -58.1368) -> (-90.9006, -58.1234) projected
  line L2424 (-90.9006, -58.1234) -> (-90.8681, -58.1107) projected
  line L2425 (-90.8681, -58.1107) -> (-90.8354, -58.0984) projected
  line L2426 (-90.8354, -58.0984) -> (-90.8025, -58.0868) projected
  line L2427 (-90.8025, -58.0868) -> (-90.7694, -58.0757) projected
  line L2428 (-90.7694, -58.0757) -> (-90.7362, -58.0652) projected
  line L2429 (-90.7362, -58.0652) -> (-90.7027, -58.0553) projected
  line L2430 (-90.7027, -58.0553) -> (-90.669, -58.046) projected
  line L2431 (-90.669, -58.046) -> (-90.6353, -58.0372) projected
  line L2432 (-90.6353, -58.0372) -> (-90.6013, -58.0291) projected
  line L2433 (-90.6013, -58.0291) -> (-90.5672, -58.0215) projected
  line L2434 (-90.5672, -58.0215) -> (-90.533, -58.0146) projected
  line L2435 (-90.533, -58.0146) -> (-90.4987, -58.0082) projected
  line L2436 (-90.4987, -58.0082) -> (-90.4643, -58.0024) projected
  line L2437 (-90.4643, -58.0024) -> (-90.4298, -57.9973) projected
  line L2438 (-90.4298, -57.9973) -> (-90.3951, -57.9927) projected
  line L2439 (-90.3951, -57.9927) -> (-90.3605, -57.9888) projected
  line L2440 (-90.3605, -57.9888) -> (-90.3257, -57.9854) projected
  line L2441 (-90.3257, -57.9854) -> (-90.2909, -57.9827) projected
  line L2442 (-90.2909, -57.9827) -> (-90.2561, -57.9806) projected
  line L2443 (-90.2561, -57.9806) -> (-90.2212, -57.979) projected
  line L2444 (-90.2212, -57.979) -> (-90.1863, -57.9781) projected
  line L2445 (-90.1863, -57.9781) -> (-90.1514, -57.9778) projected
  line L2446 (-90.1514, -57.9778) -> (-90.1165, -57.9781) projected
  line L2447 (-90.1165, -57.9781) -> (-90.0816, -57.979) projected
  line L2448 (-90.0816, -57.979) -> (-90.0467, -57.9806) projected
  line L2449 (-90.0467, -57.9806) -> (-90.0119, -57.9827) projected
  line L2450 (-90.0119, -57.9827) -> (-89.9771, -57.9854) projected
  line L2451 (-89.9771, -57.9854) -> (-89.9424, -57.9888) projected
  line L2452 (-89.9424, -57.9888) -> (-89.9077, -57.9927) projected
  line L2453 (-89.9077, -57.9927) -> (-89.8731, -57.9973) projected
  line L2454 (-89.8731, -57.9973) -> (-89.8385, -58.0024) projected
  line L2455 (-89.8385, -58.0024) -> (-89.8041, -58.0082) projected
  line L2456 (-89.8041, -58.0082) -> (-89.7698, -58.0146) projected
  line L2457 (-89.7698, -58.0146) -> (-89.7356, -58.0215) projected
  line L2458 (-89.7356, -58.0215) -> (-89.7015, -58.0291) projected
  line L2459 (-89.7015, -58.0291) -> (-89.6676, -58.0372) projected
  line L2460 (-89.6676, -58.0372) -> (-89.6338, -58.046) projected
  line L2461 (-89.6338, -58.046) -> (-89.6001, -58.0553) projected
  line L2462 (-89.6001, -58.0553) -> (-89.5667, -58.0652) projected
  line L2463 (-89.5667, -58.0652) -> (-89.5334, -58.0757) projected
  line L2464 (-89.5334, -58.0757) -> (-89.5003, -58.0868) projected
  line L2465 (-89.5003, -58.0868) -> (-89.4674, -58.0984) projected
  line L2466 (-89.4674, -58.0984) -> (-89.4347, -58.1107) projected
  line L2467 (-89.4347, -58.1107) -> (-89.4022, -58.1234) projected
  line L2468 (-89.4022, -58.1234) -> (-89.3699, -58.1368) projected
  line L2469 (-89.3699, -58.1368) -> (-89.3379, -58.1507) projected
  line L2470 (-89.3379, -58.1507) -> (-89.3062, -58.1652) projected
  line L2471 (-89.3062, -58.1652) -> (-89.2747, -58.1802) projected
  line L2472 (-89.2747, -58.1802) -> (-89.2434, -58.1958) projected
  line L2473 (-89.2434, -58.1958) -> (-89.2125, -58.2119) projected
  line L2474 (-89.2125, -58.2119) -> (-89.1818, -58.2286) projected
  line L2475 (-89.1818, -58.2286) -> (-89.1514, -58.2458) projected
  line L2476 (-89.1514, -58.2458) -> (-89.1213, -58.2635) projected
  line L2477 (-89.1213, -58.2635) -> (-89.0916, -58.2817) projected
  line L2478 (-89.0916, -58.2817) -> (-89.0621, -58.3005) projected
  line L2479 (-89.0621, -58.3005) -> (-89.033, -58.3197) projected
  line L2480 (-89.033, -58.3197) -> (-89.0043, -58.3395) projected
  line L2481 (-89.0043, -58.3395) -> (-88.9758, -58.3598) projected
  line L2482 (-88.9758, -58.3598) -> (-88.9478, -58.3805) projected
  line L2483 (-88.9478, -58.3805) -> (-88.9201, -58.4018) projected
  line L2484 (-88.9201, -58.4018) -> (-88.8928, -58.4235) projected
  line L2485 (-88.8928, -58.4235) -> (-88.8658, -58.4457) projected
  line L2486 (-88.8658, -58.4457) -> (-88.8393, -58.4684) projected
  line L2487 (-88.8393, -58.4684) -> (-88.8132, -58.4915) projected
  line L2488 (-88.8132, -58.4915) -> (-88.7874, -58.5151) projected
  line L2489 (-88.7874, -58.5151) -> (-88.7621, -58.5391) projected
  line L2490 (-88.7621, -58.5391) -> (-88.7372, -58.5636) projected
  line L2491 (-88.7372, -58.5636) -> (-88.7127, -58.5885) projected
  line L2492 (-88.7127, -58.5885) -> (-88.6887, -58.6138) projected
  line L2493 (-88.6887, -58.6138) -> (-88.6651, -58.6396) projected
  line L2494 (-88.6651, -58.6396) -> (-88.642, -58.6657) projected
  line L2495 (-88.642, -58.6657) -> (-88.6193, -58.6922) projected
  line L2496 (-88.6193, -58.6922) -> (-88.5971, -58.7192) projected
  line L2497 (-88.5971, -58.7192) -> (-88.5754, -58.7465) projected
  line L2498 (-88.5754, -58.7465) -> (-88.5541, -58.7742) projected
  line L2499 (-88.5541, -58.7742) -> (-88.5334, -58.8022) projected
  line L2500 (-88.5334, -58.8022) -> (-88.5131, -58.8307) projected
  line L2501 (-88.5131, -58.8307) -> (-88.4933, -58.8594) projected
  line L2502 (-88.4933, -58.8594) -> (-88.4741, -58.8885) projected
  line L2503 (-88.4741, -58.8885) -> (-88.4553, -58.918) projected
  line L2504 (-88.4553, -58.918) -> (-88.4371, -58.9477) projected
  line L2505 (-88.4371, -58.9477) -> (-88.4194, -58.9778) projected
  line L2506 (-88.4194, -58.9778) -> (-88.4022, -59.0082) projected
  line L2507 (-88.4022, -59.0082) -> (-88.3855, -59.0389) projected
  line L2508 (-88.3855, -59.0389) -> (-88.3694, -59.0698) projected
  line L2509 (-88.3694, -59.0698) -> (-88.3538, -59.1011) projected
  line L2510 (-88.3538, -59.1011) -> (-88.3388, -59.1326) projected
  line L2511 (-88.3388, -59.1326) -> (-88.3243, -59.1643) projected
  line L2512 (-88.3243, -59.1643) -> (-88.3104, -59.1963) projected
  line L2513 (-88.3104, -59.1963) -> (-88.297, -59.2286) projected
  line L2514 (-88.297, -59.2286) -> (-88.2843, -59.2611) projected
  line L2515 (-88.2843, -59.2611) -> (-88.272, -59.2938) projected
  line L2516 (-88.272, -59.2938) -> (-88.2604, -59.3267) projected
  line L2517 (-88.2604, -59.3267) -> (-88.2493, -59.3598) projected
  line L2518 (-88.2493, -59.3598) -> (-88.2388, -59.3931) projected
  line L2519 (-88.2388, -59.3931) -> (-88.2289, -59.4265) projected
  line L2520 (-88.2289, -59.4265) -> (-88.2196, -59.4602) projected
  line L2521 (-88.2196, -59.4602) -> (-88.2108, -59.494) projected
  line L2522 (-88.2108, -59.494) -> (-88.2027, -59.5279) projected
  line L2523 (-88.2027, -59.5279) -> (-88.1951, -59.562) projected
  line L2524 (-88.1951, -59.562) -> (-88.1882, -59.5962) projected
  line L2525 (-88.1882, -59.5962) -> (-88.1818, -59.6305) projected
  line L2526 (-88.1818, -59.6305) -> (-88.176, -59.6649) projected
  line L2527 (-88.176, -59.6649) -> (-88.1709, -59.6995) projected
  line L2528 (-88.1709, -59.6995) -> (-88.1663, -59.7341) projected
  line L2529 (-88.1663, -59.7341) -> (-88.1624, -59.7688) projected
  line L2530 (-88.1624, -59.7688) -> (-88.159, -59.8035) projected
  line L2531 (-88.159, -59.8035) -> (-88.1563, -59.8383) projected
  line L2532 (-88.1563, -59.8383) -> (-88.1542, -59.8731) projected
  line L2533 (-88.1542, -59.8731) -> (-88.1526, -59.908) projected
  line L2534 (-88.1526, -59.908) -> (-88.1517, -59.9429) projected
  line L2535 (-88.1517, -59.9429) -> (-88.1514, -59.9778) projected
  line L2536 (-88.1563, 60.1617) -> (-88.1542, 60.1269) projected
  line L2537 (-88.1542, 60.1269) -> (-88.1526, 60.092) projected
  line L2538 (-88.1526, 60.092) -> (-88.1517, 60.0571) projected
  line L2539 (-88.1517, 60.0571) -> (-88.1514, 60.0222) projected
  line L2540 (-88.1514, 60.0222) -> (-88.1517, 59.9873) projected
  line L2541 (-88.1517, 59.9873) -> (-88.1526, 59.9524) projected
  line L2542 (-88.1526, 59.9524) -> (-88.1542, 59.9175) projected
  line L2543 (-88.1542, 59.9175) -> (-88.1563, 59.8827) projected
  line L2544 (-88.1563, 59.8827) -> (-88.159, 59.8479) projected
  line L2545 (-88.159, 59.8479) -> (-88.1624, 59.8131) projected
  line L2546 (-88.1624, 59.8131) -> (-88.1663, 59.7785) projected
  line L2547 (-88.1663, 59.7785) -> (-88.1709, 59.7439) projected
  line L2548 (-88.1709, 59.7439) -> (-88.176, 59.7093) projected
  line L2549 (-88.176, 59.7093) -> (-88.1818, 59.6749) projected
  line L2550 (-88.1818, 59.6749) -> (-88.1882, 59.6406) projected
  line L2551 (-88.1882, 59.6406) -> (-88.1951, 59.6064) projected
  line L2552 (-88.1951, 59.6064) -> (-88.2027, 59.5723) projected
  line L2553 (-88.2027, 59.5723) -> (-88.2108, 59.5384) projected
  line L2554 (-88.2108, 59.5384) -> (-88.2196, 59.5046) projected
  line L2555 (-88.2196, 59.5046) -> (-88.2289, 59.4709) projected
  line L2556 (-88.2289, 59.4709) -> (-88.2388, 59.4375) projected
  line L2557 (-88.2388, 59.4375) -> (-88.2493, 59.4042) projected
  line L2558 (-88.2493, 59.4042) -> (-88.2604, 59.3711) projected
  line L2559 (-88.2604, 59.3711) -> (-88.272, 59.3382) projected
  line L2560 (-88.272, 59.3382) -> (-88.2843, 59.3055) projected
  line L2561 (-88.2843, 59.3055) -> (-88.297, 59.273) projected
  line L2562 (-88.297, 59.273) -> (-88.3104, 59.2407) projected
  line L2563 (-88.3104, 59.2407) -> (-88.3243, 59.2087) projected
  line L2564 (-88.3243, 59.2087) -> (-88.3388, 59.177) projected
  line L2565 (-88.3388, 59.177) -> (-88.3538, 59.1455) projected
  line L2566 (-88.3538, 59.1455) -> (-88.3694, 59.1142) projected
  line L2567 (-88.3694, 59.1142) -> (-88.3855, 59.0833) projected
  line L2568 (-88.3855, 59.0833) -> (-88.4022, 59.0526) projected
  line L2569 (-88.4022, 59.0526) -> (-88.4194, 59.0222) projected
  line L2570 (-88.4194, 59.0222) -> (-88.4371, 58.9921) projected
  line L2571 (-88.4371, 58.9921) -> (-88.4553, 58.9624) projected
  line L2572 (-88.4553, 58.9624) -> (-88.4741, 58.9329) projected
  line L2573 (-88.4741, 58.9329) -> (-88.4933, 58.9038) projected
  line L2574 (-88.4933, 58.9038) -> (-88.5131, 58.8751) projected
  line L2575 (-88.5131, 58.8751) -> (-88.5334, 58.8466) projected
  line L2576 (-88.5334, 58.8466) -> (-88.5541, 58.8186) projected
  line L2577 (-88.5541, 58.8186) -> (-88.5754, 58.7909) projected
  line L2578 (-88.5754, 58.7909) -> (-88.5971, 58.7636) projected
  line L2579 (-88.5971, 58.7636) -> (-88.6193, 58.7366) projected
  line L2580 (-88.6193, 58.7366) -> (-88.642, 58.7101) projected
  line L2581 (-88.642, 58.7101) -> (-88.6651, 58.6839) projected
  line L2582 (-88.6651, 58.6839) -> (-88.6887, 58.6582) projected
  line L2583 (-88.6887, 58.6582) -> (-88.7127, 58.6329) projected
  line L2584 (-88.7127, 58.6329) -> (-88.7372, 58.608) projected
  line L2585 (-88.7372, 58.608) -> (-88.7621, 58.5835) projected
  line L2586 (-88.7621, 58.5835) -> (-88.7874, 58.5595) projected
  line L2587 (-88.7874, 58.5595) -> (-88.8132, 58.5359) projected
  line L2588 (-88.8132, 58.5359) -> (-88.8393, 58.5128) projected
  line L2589 (-88.8393, 58.5128) -> (-88.8658, 58.4901) projected
  line L2590 (-88.8658, 58.4901) -> (-88.8928, 58.4679) projected
  line L2591 (-88.8928, 58.4679) -> (-88.9201, 58.4462) projected
  line L2592 (-88.9201, 58.4462) -> (-88.9478, 58.4249) projected
  line L2593 (-88.9478, 58.4249) -> (-88.9758, 58.4042) projected
  line L2594 (-88.9758, 58.4042) -> (-89.0043, 58.3839) projected
  line L2595 (-89.0043, 58.3839) -> (-89.033, 58.3641) projected
  line L2596 (-89.033, 58.3641) -> (-89.0621, 58.3449) projected
  line L2597 (-89.0621, 58.3449) -> (-89.0916, 58.3261) projected
  line L2598 (-89.0916, 58.3261) -> (-89.1213, 58.3079) projected
  line L2599 (-89.1213, 58.3079) -> (-89.1514, 58.2902) projected
  line L2600 (-89.1514, 58.2902) -> (-89.1818, 58.273) projected
  line L2601 (-89.1818, 58.273) -> (-89.2125, 58.2563) projected
  line L2602 (-89.2125, 58.2563) -> (-89.2434, 58.2402) projected
  line L2603 (-89.2434, 58.2402) -> (-89.2747, 58.2246) projected
  line L2604 (-89.2747, 58.2246) -> (-89.3062, 58.2096) projected
  line L2605 (-89.3062, 58.2096) -> (-89.3379, 58.1951) projected
  line L2606 (-89.3379, 58.1951) -> (-89.3699, 58.1812) projected
  line L2607 (-89.3699, 58.1812) -> (-89.4022, 58.1678) projected
  line L2608 (-89.4022, 58.1678) -> (-89.4347, 58.155) projected
  line L2609 (-89.4347, 58.155) -> (-89.4674, 58.1428) projected
  line L2610 (-89.4674, 58.1428) -> (-89.5003, 58.1312) projected
  line L2611 (-89.5003, 58.1312) -> (-89.5334, 58.1201) projected
  line L2612 (-89.5334, 58.1201) -> (-89.5667, 58.1096) projected
  line L2613 (-89.5667, 58.1096) -> (-89.6001, 58.0997) projected
  line L2614 (-89.6001, 58.0997) -> (-89.6338, 58.0904) projected
  line L2615 (-89.6338, 58.0904) -> (-89.6676, 58.0816) projected
  line L2616 (-89.6676, 58.0816) -> (-89.7015, 58.0735) projected
  line L2617 (-89.7015, 58.0735) -> (-89.7356, 58.0659) projected
  line L2618 (-89.7356, 58.0659) -> (-89.7698, 58.059) projected
  line L2619 (-89.7698, 58.059) -> (-89.8041, 58.0526) projected
  line L2620 (-89.8041, 58.0526) -> (-89.8385, 58.0468) projected
  line L2621 (-89.8385, 58.0468) -> (-89.8731, 58.0417) projected
  line L2622 (-89.8731, 58.0417) -> (-89.9077, 58.0371) projected
  line L2623 (-89.9077, 58.0371) -> (-89.9424, 58.0332) projected
  line L2624 (-89.9424, 58.0332) -> (-89.9771, 58.0298) projected
  line L2625 (-89.9771, 58.0298) -> (-90.0119, 58.0271) projected
  line L2626 (-90.0119, 58.0271) -> (-90.0467, 58.0249) projected
  line L2627 (-90.0467, 58.0249) -> (-90.0816, 58.0234) projected
  line L2628 (-90.0816, 58.0234) -> (-90.1165, 58.0225) projected
  line L2629 (-90.1165, 58.0225) -> (-90.1514, 58.0222) projected
  line L2630 (-90.1514, 58.0222) -> (-90.1863, 58.0225) projected
  line L2631 (-90.1863, 58.0225) -> (-90.2212, 58.0234) projected
  line L2632 (-90.2212, 58.0234) -> (-90.2561, 58.0249) projected
  line L2633 (-90.2561, 58.0249) -> (-90.2909, 58.0271) projected
  line L2634 (-90.2909, 58.0271) -> (-90.3257, 58.0298) projected
  line L2635 (-90.3257, 58.0298) -> (-90.3605, 58.0332) projected
  line L2636 (-90.3605, 58.0332) -> (-90.3951, 58.0371) projected
  line L2637 (-90.3951, 58.0371) -> (-90.4298, 58.0417) projected
  line L2638 (-90.4298, 58.0417) -> (-90.4643, 58.0468) projected
  line L2639 (-90.4643, 58.0468) -> (-90.4987, 58.0526) projected
  line L2640 (-90.4987, 58.0526) -> (-90.533, 58.059) projected
  line L2641 (-90.533, 58.059) -> (-90.5672, 58.0659) projected
  line L2642 (-90.5672, 58.0659) -> (-90.6013, 58.0735) projected
  line L2643 (-90.6013, 58.0735) -> (-90.6353, 58.0816) projected
  line L2644 (-90.6353, 58.0816) -> (-90.669, 58.0904) projected
  line L2645 (-90.669, 58.0904) -> (-90.7027, 58.0997) projected
  line L2646 (-90.7027, 58.0997) -> (-90.7362, 58.1096) projected
  line L2647 (-90.7362, 58.1096) -> (-90.7694, 58.1201) projected
  line L2648 (-90.7694, 58.1201) -> (-90.8025, 58.1312) projected
  line L2649 (-90.8025, 58.1312) -> (-90.8354, 58.1428) projected
  line L2650 (-90.8354, 58.1428) -> (-90.8681, 58.155) projected
  line L2651 (-90.8681, 58.155) -> (-90.9006, 58.1678) projected
  line L2652 (-90.9006, 58.1678) -> (-90.9329, 58.1812) projected
  line L2653 (-90.9329, 58.1812) -> (-90.9649, 58.1951) projected
  line L2654 (-90.9649, 58.1951) -> (-90.9966, 58.2096) projected
  line L2655 (-90.9966, 58.2096) -> (-91.0282, 58.2246) projected
  line L2656 (-91.0282, 58.2246) -> (-91.0594, 58.2402) projected
  line L2657 (-91.0594, 58.2402) -> (-91.0904, 58.2563) projected
  line L2658 (-91.0904, 58.2563) -> (-91.121, 58.273) projected
  line L2659 (-91.121, 58.273) -> (-91.1514, 58.2902) projected
  line L2660 (-91.1514, 58.2902) -> (-91.1815, 58.3079) projected
  line L2661 (-91.1815, 58.3079) -> (-91.2112, 58.3261) projected
  line L2662 (-91.2112, 58.3261) -> (-91.2407, 58.3449) projected
  line L2663 (-91.2407, 58.3449) -> (-91.2698, 58.3641) projected
  line L2664 (-91.2698, 58.3641) -> (-91.2986, 58.3839) projected
  line L2665 (-91.2986, 58.3839) -> (-91.327, 58.4042) projected
  line L2666 (-91.327, 58.4042) -> (-91.355, 58.4249) projected
  line L2667 (-91.355, 58.4249) -> (-91.3827, 58.4462) projected
  line L2668 (-91.3827, 58.4462) -> (-91.41, 58.4679) projected
  line L2669 (-91.41, 58.4679) -> (-91.437, 58.4901) projected
  line L2670 (-91.437, 58.4901) -> (-91.4635, 58.5128) projected
  line L2671 (-91.4635, 58.5128) -> (-91.4897, 58.5359) projected
  line L2672 (-91.4897, 58.5359) -> (-91.5154, 58.5595) projected
  line L2673 (-91.5154, 58.5595) -> (-91.5407, 58.5835) projected
  line L2674 (-91.5407, 58.5835) -> (-91.5656, 58.608) projected
  line L2675 (-91.5656, 58.608) -> (-91.5901, 58.6329) projected
  line L2676 (-91.5901, 58.6329) -> (-91.6141, 58.6582) projected
  line L2677 (-91.6141, 58.6582) -> (-91.6377, 58.6839) projected
  line L2678 (-91.6377, 58.6839) -> (-91.6608, 58.7101) projected
  line L2679 (-91.6608, 58.7101) -> (-91.6835, 58.7366) projected
  line L2680 (-91.6835, 58.7366) -> (-91.7057, 58.7636) projected
  line L2681 (-91.7057, 58.7636) -> (-91.7274, 58.7909) projected
  line L2682 (-91.7274, 58.7909) -> (-91.7487, 58.8186) projected
  line L2683 (-91.7487, 58.8186) -> (-91.7694, 58.8466) projected
  line L2684 (-91.7694, 58.8466) -> (-91.7897, 58.8751) projected
  line L2685 (-91.7897, 58.8751) -> (-91.8095, 58.9038) projected
  line L2686 (-91.8095, 58.9038) -> (-91.8287, 58.9329) projected
  line L2687 (-91.8287, 58.9329) -> (-91.8475, 58.9624) projected
  line L2688 (-91.8475, 58.9624) -> (-91.8657, 58.9921) projected
  line L2689 (-91.8657, 58.9921) -> (-91.8835, 59.0222) projected
  line L2690 (-91.8835, 59.0222) -> (-91.9006, 59.0526) projected
  line L2691 (-91.9006, 59.0526) -> (-91.9173, 59.0833) projected
  line L2692 (-91.9173, 59.0833) -> (-91.9334, 59.1142) projected
  line L2693 (-91.9334, 59.1142) -> (-91.949, 59.1455) projected
  line L2694 (-91.949, 59.1455) -> (-91.964, 59.177) projected
  line L2695 (-91.964, 59.177) -> (-91.9785, 59.2087) projected
  line L2696 (-91.9785, 59.2087) -> (-91.9924, 59.2407) projected
  line L2697 (-91.9924, 59.2407) -> (-92.0058, 59.273) projected
  line L2698 (-92.0058, 59.273) -> (-92.0186, 59.3055) projected
  line L2699 (-92.0186, 59.3055) -> (-92.0308, 59.3382) projected
  line L2700 (-92.0308, 59.3382) -> (-92.0424, 59.3711) projected
  line L2701 (-92.0424, 59.3711) -> (-92.0535, 59.4042) projected
  line L2702 (-92.0535, 59.4042) -> (-92.064, 59.4375) projected
  line L2703 (-92.064, 59.4375) -> (-92.0739, 59.4709) projected
  line L2704 (-92.0739, 59.4709) -> (-92.0833, 59.5046) projected